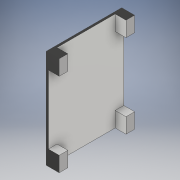
# Autodesk Inventor part: planche
Saved by Autodesk Inventor 2017 (Build 210142000, 142)
## iProperties
Created: 2018-11-08
Part Number: planche
Material: Generic
Document SubType Name: Modeling
Designer: Antoine Blaud
Density: 1 g/cm^3
Appearance: Default
Author: Antoine Blaud
Autodesk Inventor part; units mm, degrees
ref_plane "YZ Plane" through (0, 0, 0) normal (1, 0, 0) x (0, 1, 0)
ref_plane "XZ Plane" through (0, 0, 0) normal (0, 1, 0) x (-1, 0, 0)
ref_plane "XY Plane" through (0, 0, 0) normal (0, 0, 1) x (1, 0, 0)
sketch "Sketch1" plane through (0, 0, 0) normal (1, 0, 0) x (0, 1, 0)
  line L0 (146.5161, -47.399) -> (-150.4839, -47.399)
  line L1 (-150.4839, -47.399) -> (-150.4839, -257.399)
  line L2 (-150.4839, -257.399) -> (146.5161, -257.399)
  line L3 (146.5161, -257.399) -> (146.5161, -47.399)
  line L4 (176.5161, -17.399) -> (-180.4839, -17.399)
  line L5 (-180.4839, -17.399) -> (-180.4839, -287.399)
  line L6 (-180.4839, -287.399) -> (176.5161, -287.399)
  line L7 (176.5161, -287.399) -> (176.5161, -17.399)
  point P0 (0, 0)
  dimension "d0" = 297
  dimension "d1" = 210
  dimension "d2" = 30
  dimension "d3" = 30
  dimension "d4" = 30
  dimension "d5" = 30
  constraints: 16 end point, 4 parallel, 2 horizontal, 2 perpendicular
  measures "d0" distance of L1.end L2.end
  measures "d1" distance of L0.end L1.end
  measures "d2" distance between parallel lines of L7 L3
  measures "d3" distance between parallel lines of L1 L5
  measures "d4" distance between parallel lines of L6 L2
  measures "d5" distance between parallel lines of L4 L0
extrude "Extrusion1" add sketch "Sketch1" along normal blind 10 contours L3 L2 L1 L0
sketch "Sketch2" plane through (10, 0, 0) normal (1, 0, 0) x (0, 0, -1)
  point P0 (0, 0)
sketch "Sketch3" plane through (10, 0, 0) normal (1, 0, 0) x (0, 0, -1)
  line L0 (17.899, 176.0161) -> (286.899, 176.0161)
  line L1 (286.899, 176.0161) -> (286.899, -179.9839)
  line L2 (286.899, -179.9839) -> (17.899, -179.9839)
  line L3 (17.899, -179.9839) -> (17.899, 176.0161)
  line L4 (257.399, 146.5161) -> (47.399, 146.5161) projected
  line L5 (47.399, -150.4839) -> (257.399, -150.4839) projected
  line L6 (47.399, 146.5161) -> (47.399, -150.4839) projected
  line L7 (257.399, -150.4839) -> (257.399, 146.5161) projected
  point P0 (0, 0)
  dimension "d8" = 29.5
  dimension "d9" = 29.5
  dimension "d10" = 29.5
  dimension "d11" = 29.5
  constraints: 8 end point, 2 parallel, 1 horizontal, 1 perpendicular
  measures "d8" distance between parallel lines of L0 L4
  measures "d9" distance between parallel lines of L2 L5
  measures "d10" distance between parallel lines of L3 L6
  measures "d11" distance between parallel lines of L1 L7
extrude "Extrusion2" add sketch "Sketch3" against normal blind 14
sketch "Sketch4" plane through (10, 176.0161, -17.899) normal (0, 1, 0) x (1, 0, 0)
  point P0 (-10, -17.899)
sketch "Sketch5" plane through (0, 0, 0) normal (-1, 0, 0) x (0, 0, 1)
  point P0 (0, 0)
sketch "Sketch6" plane through (0, 0, 0) normal (-1, 0, 0) x (0, 0, 1)
  line L0 (-257.399, -150.4839) -> (-257.399, 146.5161) projected
  circle A0 centre (-257.399, -1.9839) radius 23.7269
  line L1 (-257.399, -25.7108) -> (-257.399, 21.7431)
  point P0 (0, 0)
  constraints: 2 end point, 2 point on circle, 2 point on line, 1 centre point, 1 midpoint
extrude "Extrusion3" cut sketch "Sketch6" along normal blind 10 and the other way blind 3 contours A0 L0 picked at (-265.2503, -2.9372)
fillet "Fillet1" radius 3 1 edges at (3, -1.9839, -281.1259)
sketch "Sketch7" plane through (0, 0, 0) normal (-1, 0, 0) x (0, 0, 1)
  line L0 (-326.899, -229.9839) -> (22.101, -229.9839)
  line L1 (22.101, -229.9839) -> (22.101, 226.5161)
  line L2 (22.101, 226.5161) -> (-326.899, 226.5161)
  line L3 (-326.899, 226.5161) -> (-326.899, -229.9839)
  line L4 (-257.399, 146.5161) -> (-47.399, 146.5161) projected
  line L5 (-17.899, -179.9839) -> (-17.899, 176.0161) projected
  line L6 (-286.899, 176.0161) -> (-286.899, -179.9839) projected
  line L7 (-286.899, -179.9839) -> (-17.899, -179.9839) projected
  point P0 (0, 0)
  dimension "d19" = 80
  dimension "d20" = 40
  dimension "d21" = 40
  dimension "d22" = 50
  constraints: 8 end point, 2 parallel, 1 horizontal, 1 perpendicular
  measures "d19" distance between parallel lines of L2 L4
  measures "d20" distance between parallel lines of L1 L5
  measures "d21" distance between parallel lines of L6 L3
  measures "d22" distance between parallel lines of L0 L7
extrude "Extrusion4" add sketch "Sketch7" against normal blind 10
sketch "Sketch10" plane through (0, 0, 0) normal (-1, 0, 0) x (0, 0, 1)
  circle A0 centre (0, 176.2762) radius 12.5
  line L0 (-326.899, 226.5161) -> (-326.899, -229.9839) projected
  line L1 (-326.899, 0) -> (22.101, 0)
  line L2 (22.101, -229.9839) -> (22.101, 226.5161) projected
  line L3 (-326.899, 176.2762) -> (22.101, 176.2762)
  line L4 (-326.899, -179.9839) -> (22.101, -179.9839)
  line L5 (0, 176.2762) -> (0, -179.9839)
  circle A1 centre (0, -179.9839) radius 12.5
  line L6 (-17.899, -179.9839) -> (-17.899, 176.0161) projected
  circle A2 centre (-304.798, -179.9839) radius 12.5
  line L7 (-286.899, 176.0161) -> (-286.899, -179.9839) projected
  line L8 (-304.798, -179.9839) -> (-304.798, 176.2762)
  circle A3 centre (-304.798, 176.2762) radius 12.5
  point P0 (0, 0)
  dimension "d26" = 25
  dimension "d27" = 25
  dimension "d28" = 17.899
  dimension "d29" = 25
  dimension "d30" = 17.899
  dimension "d31" = 25
  constraints: 10 end point, 9 point on line, 4 centre point, 4 perpendicular, 2 coincident, 1 horizontal
  measures "d26" diameter of A0
  measures "d27" diameter of A1
  measures "d28" distance between parallel lines of L5 L6
  measures "d29" diameter of A2
  measures "d30" distance from line of L7 L8.start
  measures "d31" diameter of A3
extrude "Extrusion5" cut sketch "Sketch10" against normal blind 20 contours L3 A0 | A0 L5 L3 | L3 L5 A0 | A3 L8 L3 | L3 A3 | L8 A3 L3 | A1 L4 L5 | L5 L4 A1 | L4 A1 | L8 L4 A2 | A2 L4 L8 | A2 L4
sketch "Sketch11" plane through (10, 0, 0) normal (1, 0, 0) x (0, 0, -1)
  line L0 (326.899, 226.5161) -> (-22.101, 226.5161) projected
  line L1 (17.899, 226.5161) -> (-22.101, 226.5161)
  line L2 (-22.101, 226.5161) -> (-22.101, 156.5161)
  line L3 (-22.101, 156.5161) -> (17.899, 156.5161)
  line L4 (17.899, 156.5161) -> (17.899, 226.5161)
  line L5 (-22.101, -229.9839) -> (326.899, -229.9839) projected
  line L6 (17.899, -229.9839) -> (-22.101, -229.9839)
  line L7 (-22.101, -229.9839) -> (-22.101, -159.9839)
  line L8 (-22.101, -159.9839) -> (17.899, -159.9839)
  line L9 (17.899, -159.9839) -> (17.899, -229.9839)
  line L10 (326.899, 226.5161) -> (286.899, 226.5161)
  line L11 (286.899, 226.5161) -> (286.899, 156.5161)
  line L12 (286.899, 156.5161) -> (326.899, 156.5161)
  line L13 (326.899, 156.5161) -> (326.899, 226.5161)
  line L14 (326.899, -229.9839) -> (286.899, -229.9839)
  line L15 (286.899, -229.9839) -> (286.899, -159.9839)
  line L16 (286.899, -159.9839) -> (326.899, -159.9839)
  line L17 (326.899, -159.9839) -> (326.899, -229.9839)
  point P0 (0, 0)
  dimension "d34" = 40
  dimension "d35" = 70
  dimension "d36" = 40
  dimension "d37" = 70
  dimension "d38" = 70
  dimension "d39" = 40
  dimension "d40" = 70
  dimension "d41" = 40
  constraints: 32 end point, 8 parallel, 4 horizontal, 4 perpendicular, 2 point on line
  measures "d34" distance between parallel lines of L4 L2
  measures "d35" distance between parallel lines of L3 L0
  measures "d36" distance between parallel lines of L7 L9
  measures "d37" distance between parallel lines of L8 L5
  measures "d38" distance between parallel lines of L0 L12
  measures "d39" distance between parallel lines of L13 L11
  measures "d40" distance between parallel lines of L16 L14
  measures "d41" distance between parallel lines of L17 L15
extrude "Extrusion6" add sketch "Sketch11" along normal blind 50
body "Solid1"
